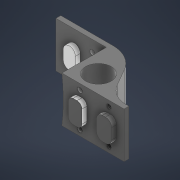
# Autodesk Inventor part: sensorbar
Saved by Autodesk Inventor 2022 (Build 260153000, 153)
## iProperties
Created: 2021-10-11
Part Number: sensorbar
Material: ABS プラスチック
Document SubType Name: Modeling
Designer: shiok
Density: 1.06 g/cm^3
Appearance: 滑らか - 白
Mass: 4.64134 g
Surface Area: 39.738 cm^2
Volume: 4.37862 cm^3
Author: shiok
Autodesk Inventor part; units mm, degrees
ref_plane "YZ Plane" through (0, 0, 0) normal (1, 0, 0) x (0, 1, 0)
ref_plane "XZ Plane" through (0, 0, 0) normal (0, 1, 0) x (-1, 0, 0)
ref_plane "XY Plane" through (0, 0, 0) normal (0, 0, 1) x (1, 0, 0)
sketch "スケッチ14" plane through (0, 0, 0) normal (0, 1, 0) x (-1, 0, 0)
  line L0 (0, -17.8) -> (-9.2265, -17.8)
  line L1 (-29, -3.2) -> (-29, 0)
  line L2 (-29, 0) -> (-9, 0)
  line L3 (0, -16.2) -> (-9, -16.2)
  line L4 (-17.8868, -12.8) -> (-21.1199, -7.2)
  line L5 (-28.0481, -3.2) -> (-29, -3.2)
  line L6 (0, -16.2) -> (0, -17.8)
  line L7 (-9, -16.2) -> (-9, 0)
  arc A0 (-17.8868, -12.8) -> (-9.2265, -17.8) centre (-9.2265, -7.8) ccw
  arc A1 (-21.1199, -7.2) -> (-28.0481, -3.2) centre (-28.0481, -11.2) ccw
  circle A2 centre (-14.7921, -7.3921) radius 4.1921
  line L8 (-14.7921, -3.2) -> (-14.7921, 0)
  line L9 (-10.6, -7.3921) -> (-9, -7.3921)
  line L10 (-18.8213, -8.5495) -> (-20.3591, -8.9913)
  point P0 (0, 0)
  point P1 (-23.4293, -3.2)
  point P2 (-15, -17.8)
  dimension "d97" = 1.6
  dimension "d99" = 3.2
  dimension "d101" = 15
  dimension "d102" = 20
  dimension "d106" = 16.2
  dimension "d119" = 9
  dimension "d129" = 1.6
  dimension "d146" = 8
  dimension "d147" = 10
  dimension "d148" = 120
  dimension "d190" = 3.2
  constraints: 22 end point, 12 point on line, 8 point on circle, 5 perpendicular, 4 tangent, 3 centre point, 2 horizontal, 2 parallel, 1 equal length
  measures "d97" distance between parallel lines of L0 L3
  measures "d99" distance between parallel lines of L5 L2
  measures "d101" distance of point (-15, -17.8) L0.start
  measures "d102" distance of L2.end L1.end
  measures "d106" distance between parallel lines of L3 L2
  measures "d119" distance of L3.start L3.end
  measures "d129" distance of L9.start L9.end
  measures "d146" radius of A1
  measures "d147" radius of A0
  measures "d148" angle of L4 L5
  measures "d190" distance of L8.start L8.end
extrude "押し出し5" add sketch "スケッチ14" along normal blind 15 contours L0 A0 L4 L10 A2 L9 L7 L3 L6 | L4 A1 L5 L1 L2 L8 A2 L10 | L9 A2 L8 L2 L7
sketch "スケッチ23" plane through (29, 0, 0) normal (0, 0, 1) x (1, 0, 0)
  line L0 (-20, 15) -> (0, 15) projected
  line L1 (0, 0) -> (-0.9519, 0) projected
  line L2 (0, 0) -> (-10, 0)
  line L3 (-10, 0) -> (-10, 15)
  line L4 (-10, 15) -> (0, 15)
  line L5 (0, 15) -> (0, 0)
  line L6 (-5.5, 11.25) -> (-5, 11.25)
  line L7 (-5, 11.25) -> (-5, 7.5) construction
  line L8 (-5, 7.5) -> (-7.5, 7.5) construction
  line L9 (-7.5, 7.5) -> (-7.5, 9.25)
  line L10 (-4.5, 11.25) -> (-5, 11.25)
  line L11 (-2.5, 7.5) -> (-2.5, 9.25)
  line L12 (-5.5, 3.75) -> (-5, 3.75)
  line L13 (-7.5, 7.5) -> (-7.5, 5.75)
  line L14 (-2.5, 7.5) -> (-2.5, 5.75)
  line L15 (-4.5, 3.75) -> (-5, 3.75)
  line L16 (-7.5, 7.5) -> (-10, 7.5) construction
  line L17 (-5, 11.25) -> (-5, 15) construction
  arc A0 (-5.5, 11.25) -> (-7.5, 9.25) centre (-5.5, 9.25) ccw
  arc A1 (-7.5, 5.75) -> (-5.5, 3.75) centre (-5.5, 5.75) ccw
  arc A2 (-4.5, 3.75) -> (-2.5, 5.75) centre (-4.5, 5.75) ccw
  arc A3 (-2.5, 9.25) -> (-4.5, 11.25) centre (-4.5, 9.25) ccw
  point P0 (-29, 0)
  point P1 (-7.5, 11.25)
  point P2 (-2.5, 11.25)
  point P3 (-7.5, 3.75)
  point P4 (-2.5, 3.75)
  dimension "d150" = 10
  dimension "d151" = 15
  dimension "d154" = 2
  constraints: 32 end point, 8 point on circle, 8 point on line, 8 tangent, 5 symmetric about line, 4 centre point, 4 collinear, 4 parallel, 3 equal radius, 2 horizontal, 2 midpoint, 2 perpendicular
  measures "d150" distance of L3.end L4.end
  measures "d151" distance of L2.end L3.end
  measures "d154" radius of A0
extrude "押し出し10" cut sketch "スケッチ23" against normal blind 1.6
sketch "スケッチ24" plane through (29, 0, -1.6) normal (0, 0, 1) x (1, 0, 0)
  line L0 (-10, 15) -> (0, 15) projected
  line L1 (-10, 0) -> (-10, 15) projected
  line L2 (0, 0) -> (-10, 0) projected
  line L3 (0, 15) -> (0, 0) projected
  line L4 (-7.5, 9.25) -> (-7.5, 5.75) projected
  arc A0 (-5.5, 11.25) -> (-7.5, 9.25) centre (-5.5, 9.25) ccw projected
  line L5 (-4.5, 11.25) -> (-5.5, 11.25) projected
  arc A1 (-2.5, 9.25) -> (-4.5, 11.25) centre (-4.5, 9.25) ccw projected
  line L6 (-2.5, 5.75) -> (-2.5, 9.25) projected
  arc A2 (-4.5, 3.75) -> (-2.5, 5.75) centre (-4.5, 5.75) ccw projected
  line L7 (-5.5, 3.75) -> (-4.5, 3.75) projected
  arc A3 (-7.5, 5.75) -> (-5.5, 3.75) centre (-5.5, 5.75) ccw projected
  arc A4 (-5.5, 11.25) -> (-7.5, 9.25) centre (-5.5, 9.25) ccw projected
  line L8 (-7.5, 9.25) -> (-7.5, 5.75) projected
  arc A5 (-7.5, 5.75) -> (-5.5, 3.75) centre (-5.5, 5.75) ccw projected
  line L9 (-5.5, 3.75) -> (-4.5, 3.75) projected
  arc A6 (-4.5, 3.75) -> (-2.5, 5.75) centre (-4.5, 5.75) ccw projected
  line L10 (-2.5, 5.75) -> (-2.5, 9.25) projected
  arc A7 (-2.5, 9.25) -> (-4.5, 11.25) centre (-4.5, 9.25) ccw projected
  line L11 (-4.5, 11.25) -> (-5.5, 11.25) projected
  line L12 (-5, 13.125) -> (-5, 15) construction
  line L13 (0, 15) -> (-0.9519, 15) construction
  line L14 (-5, 13.125) -> (-5, 11.25) construction
  line L15 (-4.5, 11.25) -> (-5.5, 11.25) construction
  line L16 (-5.5, 3.75) -> (-4.5, 3.75) construction
  line L17 (-5, 3.75) -> (-5, 1.875) construction
  line L18 (-5, 1.875) -> (-5, 0) construction
  line L19 (0, 0) -> (-0.9519, 0) construction
  point P0 (-29, 0)
  constraints: 8 end point, 5 collinear, 2 midpoint, 2 point on line, 1 perpendicular
hole "穴9" at (24, 1.875, -1.6) at (24, 13.125, -1.6) direction (0, 0, -1) diameter 1.567 end up to face face through (28.0481, 0, -11.2) facing (0, 1, 0) round with radius 8 far side no thread size "M2x0.4" class "6H" standard "ISO Metric profile"
sketch "スケッチ25" plane through (9, 0, 0) normal (0, 0, 1) x (1, 0, 0)
  line L0 (0, 0) -> (0, 15) projected
  line L1 (10, 0) -> (10, 15) projected
  arc A0 (-0.4516, 0) -> (-0.4516, 15) centre (-62.5, 7.5) ccw
  line L2 (0, 0) -> (20, 0) projected
  line L3 (0, 15) -> (20, 15) projected
  line L4 (-0.4516, 15) -> (0, 15)
  line L5 (-0.4516, 0) -> (0, 0)
  line L6 (0, 0) -> (0, 15) projected
  line L7 (0, 7.5) -> (-62.5, 7.5)
  point P0 (0, 7.5)
  dimension "d166" = 62.5
  constraints: 6 end point, 2 horizontal, 2 point on circle, 2 point on line, 1 centre point, 1 coincident, 1 midpoint, 1 tangent
  measures "d166" distance of L7.start L7.end
extrude "押し出し11" add sketch "スケッチ25" against normal up to surface contours L5 A0 L0 | A0 L4 L0 round surface about axis through (9.2265, 0, -7.8) along (0, 1, 0) radius 10 far side no
sketch "スケッチ26" plane through (9.2265, 0, -17.8) normal (0, 0, -1) x (-1, 0, 0)
  line L0 (0, 0) -> (9.2265, 0) projected
  line L1 (9.2265, 0) -> (9.2265, 15) projected
  line L2 (0, 15) -> (9.2265, 15) projected
  line L3 (0, 0) -> (0, 15) projected
  line L4 (9.2265, 0) -> (9.2265, 15) projected
  line L5 (9.2265, 7.5) -> (0, 7.5)
  line L6 (0, 0) -> (0, 15) projected
  point P0 (5.2265, 3.75)
  point P1 (5.2265, 11.25)
  dimension "d206" = 4
  dimension "d207" = 3.75
  constraints: 2 end point, 2 midpoint, 1 symmetric about line
  measures "d206" distance from line of L1 point (5.226, 3.75)
  measures "d207" distance from line of L0 point (5.226, 3.75)
hole "穴10" at (4, 3.75, -17.8) at (4, 11.25, -17.8) direction (0, 0, 1) diameter 1.567 depth 1.6 tip angle 118 thread size "M2x0.4" class "6H" standard "ISO Metric profile"
ref_plane "作業平面1" through (0, 7.5, 0) normal (0, 1, 0) x (1, 0, 0)
sketch "スケッチ28" plane through (19, 0, 0) normal (0, 0, 1) x (1, 0, 0)
  arc A0 (-10.4516, 0) -> (-10.4516, 15) centre (-72.5, 7.5) ccw projected
  line L0 (0, 0) -> (0, 15) projected
  line L1 (-9, 15) -> (-9, 0)
  line L2 (-5.15, 11.25) -> (-3.85, 11.25)
  line L3 (-2.25, 9.65) -> (-2.25, 7.5)
  line L4 (-6.75, 7.5) -> (-6.75, 9.65)
  line L5 (0, 0) -> (0, 15) projected
  line L6 (-9, 15) -> (0, 15)
  line L7 (-9, 0) -> (0, 0)
  line L8 (-9, 7.5) -> (-6.75, 7.5)
  line L9 (-2.25, 7.5) -> (0, 7.5)
  line L10 (-6.75, 7.5) -> (-4.5, 7.5)
  line L11 (-4.5, 7.5) -> (-2.25, 7.5)
  arc A1 (4.5, 11.25) -> (2.5, 9.25) centre (4.5, 9.25) ccw projected
  line L12 (2.5, 9.25) -> (2.5, 5.75) projected
  arc A2 (2.5, 5.75) -> (4.5, 3.75) centre (4.5, 5.75) ccw projected
  line L13 (4.5, 3.75) -> (5.5, 3.75) projected
  arc A3 (5.5, 3.75) -> (7.5, 5.75) centre (5.5, 5.75) ccw projected
  line L14 (7.5, 5.75) -> (7.5, 9.25) projected
  arc A4 (7.5, 9.25) -> (5.5, 11.25) centre (5.5, 9.25) ccw projected
  line L15 (5.5, 11.25) -> (4.5, 11.25) projected
  arc A5 (-5.15, 11.25) -> (-6.75, 9.65) centre (-5.15, 9.65) ccw
  arc A6 (-2.25, 9.65) -> (-3.85, 11.25) centre (-3.85, 9.65) ccw
  line L16 (-5.15, 3.75) -> (-3.85, 3.75)
  line L17 (-2.25, 5.35) -> (-2.25, 7.5)
  line L18 (-6.75, 7.5) -> (-6.75, 5.35)
  arc A7 (-6.75, 5.35) -> (-5.15, 3.75) centre (-5.15, 5.35) ccw
  arc A8 (-3.85, 3.75) -> (-2.25, 5.35) centre (-3.85, 5.35) ccw
  line L19 (0, 15) -> (-10.4516, 15) projected
  line L20 (-9, 15) -> (-10.4516, 15)
  line L21 (-10.4516, 0) -> (0, 0) projected
  line L22 (-10.4516, 15) -> (-10.4516, 0)
  line L23 (-10.4516, 0) -> (-9, 0)
  line L24 (-10.4516, 0) -> (-9, 0)
  dimension "d186" = 1
  dimension "d187" = 1.6
  constraints: 34 end point, 8 collinear, 8 point on circle, 6 symmetric about line, 4 centre point, 4 horizontal, 4 tangent, 2 midpoint, 2 parallel, 2 perpendicular, 1 equal radius, 1 vertical, 2 other
  measures "d186" distance edge to line of A0 L1
  measures "d187" radius of A5
extrude "押し出し12" cut sketch "スケッチ28" against normal blind 1.6 contours A0 L19 L1 L21 | L1 L8 L18 A7 L16 A8 L17 L9 L0 L7 | L6 L0 L9 L3 A6 L2 A5 L4 L8 L1
sketch "スケッチ29" plane through (29, 0, -1.6) normal (0, 0, 1) x (1, 0, 0)
  circle A0 centre (-5, 1.875) radius 0.7835 projected
  circle A1 centre (-5, 13.125) radius 0.7835 projected
  line L0 (-13.85, 11.25) -> (-15.15, 11.25) projected
  point P0 (-29, 0)
  point P1 (-14.5, 13.125)
  point P2 (-14.5, 1.875)
  point P3 (-14.5, 11.25)
  constraints: 2 horizontal alignment, 2 vertical alignment, 1 midpoint
hole "穴12" at (14.5, 1.875, -1.6) at (14.5, 13.125, -1.6) direction (0, 0, -1) diameter 1.567 depth 6.3 tip angle 118 thread size "M2x0.4" class "6H" standard "ISO Metric profile"
sketch "スケッチ31" plane through (0, 0, -17.8) normal (-1, 0, 0) x (0, 0, 1)
  line L0 (0, 0) -> (1.6, 0) projected
  line L1 (1.6, 0) -> (1.6, 15) projected
  line L2 (0, 0) -> (1.6, 0)
  line L3 (1.6, 0) -> (1.6, 15)
  line L4 (1.6, 15) -> (0, 15)
  line L5 (0, 15) -> (0, 0)
  point P0 (17.8, 0)
  constraints: 8 end point, 2 parallel, 1 horizontal, 1 perpendicular
extrude "押し出し13" add sketch "スケッチ31" along normal blind 8
sketch "スケッチ34" plane through (-53.5, 7.5, -16.2) normal (0, 0, 1) x (1, 0, 0)
  circle A0 centre (57.5, 3.75) radius 0.7835 projected
  circle A1 centre (57.5, -3.75) radius 0.7835 projected
  line L0 (57.5, 3.75) -> (57.5, -3.75)
  line L1 (49.5, 3.5) -> (53.5, 3.5)
  line L2 (53.5, 3.5) -> (53.5, -3.5)
  line L3 (53.5, -3.5) -> (49.5, -3.5)
  line L4 (49.5, -3.5) -> (49.5, 3.5)
  line L5 (49.5, 3.5) -> (53.5, -3.5) construction
  line L6 (49.5, -3.5) -> (53.5, 3.5) construction
  line L7 (51.5, 0) -> (57.5, 0) construction
  point P0 (53.5, -7.5)
  dimension "d208" = 6
  dimension "d209" = 7
  dimension "d210" = 4
  constraints: 16 end point, 3 midpoint, 2 parallel, 2 perpendicular, 1 horizontal, 1 vertical
  measures "d208" distance of L7.start L7.end
  measures "d209" distance of L3.end L1.start
  measures "d210" distance of L1.start L1.end
extrude "押し出し15" add sketch "スケッチ34" along normal blind 1.6 contours L1 L2 L3 L4
fillet "フィレット19" radius 2 4 edges at (0, 4, -15.4) (-4, 4, -15.4) (-4, 11, -15.4) (0, 11, -15.4)
